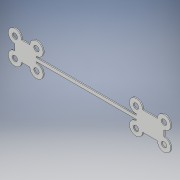
# Autodesk Inventor part: NerfMount
Saved by Autodesk Inventor 2018.3 (Build 223284000, 284)
## iProperties
Created: 2019-08-17
Part Number: NerfMount
Material: Generic
Document SubType Name: Modeling
Designer: Srinity
Density: 1 g/cm^3
Appearance: Default
Author: Srinity
Autodesk Inventor part; units mm, degrees
ref_plane "YZ Plane" through (0, 0, 0) normal (1, 0, 0) x (0, 1, 0)
ref_plane "XZ Plane" through (0, 0, 0) normal (0, 1, 0) x (-1, 0, 0)
ref_plane "XY Plane" through (0, 0, 0) normal (0, 0, 1) x (1, 0, 0)
sketch "Sketch1" plane through (0, 0, 0) normal (0, 0, 1) x (1, 0, 0)
  line L0 (169.1393, 4.2882) -> (221.6393, 4.2882)
  line L1 (221.6393, 4.2882) -> (221.6393, -32.0118)
  line L2 (221.6393, -32.0118) -> (169.1393, -32.0118)
  line L3 (169.1393, -32.0118) -> (169.1393, 4.2882)
  line L4 (-58.3607, 4.2882) -> (-17.8607, 4.2882)
  line L5 (-17.8607, 4.2882) -> (-17.8607, -32.0118)
  line L6 (-17.8607, -32.0118) -> (-58.3607, -32.0118)
  line L7 (-58.3607, -32.0118) -> (-58.3607, 4.2882)
  circle A0 centre (-58.3607, 4.2882) radius 12.5
  circle A1 centre (-58.3607, -32.0118) radius 12.5
  circle A2 centre (-17.8607, -32.0118) radius 12.5
  circle A3 centre (-17.8607, 4.2882) radius 12.5
  circle A4 centre (169.1393, 4.2882) radius 12.5
  circle A5 centre (169.1393, -32.0118) radius 12.5
  circle A6 centre (221.6393, -32.0118) radius 12.5
  circle A7 centre (221.6393, 4.2882) radius 12.5
  line L8 (-34.8317, -10.7118) -> (176.5512, -10.7118)
  line L9 (176.5512, -10.7118) -> (176.5512, -17.0118)
  line L10 (176.5512, -17.0118) -> (-34.8317, -17.0118)
  line L11 (-34.8317, -17.0118) -> (-34.8317, -10.7118)
  dimension "d0" = 36.3
  dimension "d1" = 40.5
  dimension "d2" = 52.5
  dimension "d3" = 239.5
  dimension "d4" = 25
  dimension "d5" = 15
  dimension "d6" = 15
  constraints: 24 end point, 8 centre point, 8 coincident, 7 equal radius, 6 parallel, 3 horizontal, 3 perpendicular, 1 collinear, 1 point on line
  measures "d0" distance of L4.end L5.end
  measures "d1" distance of L4.start L4.end
  measures "d2" distance of L0.start L0.end
  measures "d3" distance between parallel lines of L1 L5
  measures "d4" diameter of A3
  measures "d5" distance between parallel lines of L8 L4
  measures "d6" distance between parallel lines of L10 L6
extrude "Extrusion1" add sketch "Sketch1" along normal blind 2
sketch "Sketch2" plane through (0, 0, 2) normal (0, 0, 1) x (1, 0, 0)
  circle A0 centre (-58.3607, 4.2882) radius 5
  circle A1 centre (-58.3607, -32.0118) radius 5
  circle A2 centre (-17.8607, -32.0118) radius 5
  circle A3 centre (-17.8607, 4.2882) radius 5
  circle A4 centre (169.1393, 4.2882) radius 5
  circle A5 centre (169.1393, -32.0118) radius 5
  circle A6 centre (221.6393, -32.0118) radius 5
  circle A7 centre (221.6393, 4.2882) radius 5
  arc A8 (-45.8607, 4.2882) -> (-58.3607, -8.2118) centre (-58.3607, 4.2882) ccw projected
  arc A9 (-17.8607, -8.2118) -> (-30.3607, 4.2882) centre (-17.8607, 4.2882) ccw projected
  arc A10 (-58.3607, -19.5118) -> (-45.8607, -32.0118) centre (-58.3607, -32.0118) ccw projected
  arc A11 (-30.3607, -32.0118) -> (-17.8607, -19.5118) centre (-17.8607, -32.0118) ccw projected
  arc A12 (169.1393, -19.5118) -> (181.6393, -32.0118) centre (169.1393, -32.0118) ccw projected
  arc A13 (181.6393, 4.2882) -> (169.1393, -8.2118) centre (169.1393, 4.2882) ccw projected
  arc A14 (221.6393, -8.2118) -> (209.1393, 4.2882) centre (221.6393, 4.2882) ccw projected
  arc A15 (209.1393, -32.0118) -> (221.6393, -19.5118) centre (221.6393, -32.0118) ccw projected
  point P0 (0, 0)
  dimension "d9" = 10
  constraints: 8 centre point, 8 concentric, 7 equal radius
  measures "d9" diameter of A0
extrude "Extrusion2" cut sketch "Sketch2" against normal blind 2
equation "\"d6\" = d5"
body "Solid1"
